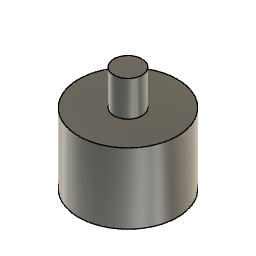
assembly v2 (Autodesk Fusion 360 archive; units mm, degrees)
design "motor1"
Autodesk Fusion 360 part; units mm, degrees
sketch "Sketch1" plane through (0, 0, 0) normal (0, 0, 1) x (1, 0, 0)
  circle A0 centre (0, 0) radius 35
  dimension "d1" = 70
  constraint coincident A0.centre origin
  measures "d1" diameter of A0
extrude "Extrude1" add sketch "Sketch1" along normal blind 50
sketch "Sketch2" plane through (0, 0, 50) normal (0, 0, 1) x (-1, 0, 0)
  circle A0 centre (0, 0) radius 35
  circle A1 centre (0, 0) radius 10
  dimension "d4" = 20
  constraint coincident A0.centre A1.centre
  measures "d4" diameter of A1
extrude "Extrude2" add sketch "Sketch2" along normal blind 25 contours A1

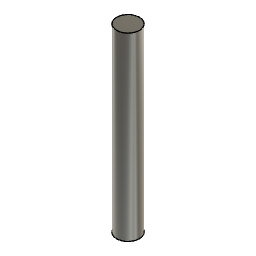
design "crod1"
Autodesk Fusion 360 part; units mm, degrees
sketch "Sketch1" plane through (0, 0, 0) normal (0, 0, 1) x (1, 0, 0)
  circle A0 centre (-0.4902, 0) radius 3
  dimension "d1" = 6
  measures "d1" diameter of A0
extrude "Extrude1" add sketch "Sketch1" along normal blind 47.5

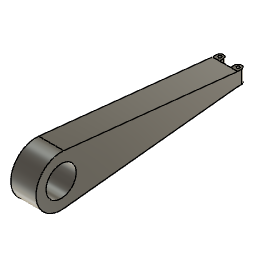
design "arm2"
Autodesk Fusion 360 part; units mm, degrees
sketch "Sketch1" plane through (0, 0, 0) normal (1, 0, 0) x (0, 1, 0)
  circle A0 centre (0, 0) radius 30
  line L0 (5.2264, 49.7261) -> (351.0282, 13.3809)
  line L1 (5.2991, -49.7184) -> (351.0282, -12.87)
  line L2 (351.0282, 13.3809) -> (351.0282, -12.87)
  arc A1 (5.2264, 49.7261) -> (5.2991, -49.7184) centre (0, 0) ccw
  dimension "d1" = 100
  dimension "d2" = 60
  constraint coincident A0.centre A1.centre
  constraint tangent L0 A1
  constraint vertical L2
  measures "d1" diameter of A1
  measures "d2" diameter of A0
extrude "Extrude1" add sketch "Sketch1" along normal blind 50
sketch "Sketch2" plane through (0, 0, 0) normal (0, 0, 1) x (1, 0, 0)
  line L0 (50, 351) -> (36, 351)
  line L1 (36, 351) -> (36, 359)
  line L2 (50, 359) -> (50, 351)
  circle A0 centre (43, 359) radius 3
  line L3 (0, 351) -> (14, 351)
  line L4 (14, 351) -> (14, 359)
  line L5 (0, 359) -> (0, 351)
  circle A1 centre (7, 359) radius 3
  arc A2 (50, 359) -> (36, 359) centre (43, 359) ccw
  arc A3 (14, 359) -> (0, 359) centre (7, 359) ccw
  dimension "d9" = 6
  dimension "d12" = 6
  constraint horizontal L0
  constraint vertical L1
  constraint vertical L2
  constraint concentric A0 A2
  constraint horizontal L3
  constraint vertical L4
  constraint vertical L5
  constraint concentric A1 A3
  measures "d9" diameter of A0
  measures "d12" diameter of A1
extrude "Extrude2" add sketch "Sketch2" along normal blind 13.355 and the other way blind 13.1255
equation "d13 = ( 26.71 / 2 ) * 1 mm"
equation "d15 = ( 26.251 / 2 ) * 1 mm"

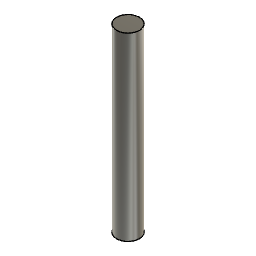
design "crod2"
Autodesk Fusion 360 part; units mm, degrees
sketch "Sketch1" plane through (0, 0, 0) normal (0, 0, 1) x (1, 0, 0)
  circle A0 centre (0, 0) radius 3
  dimension "d1" = 6
  constraint coincident A0.centre origin
  measures "d1" diameter of A0
extrude "Extrude1" add sketch "Sketch1" along normal blind 47.5

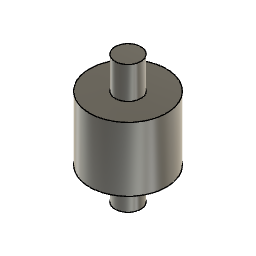
design "motor3"
Autodesk Fusion 360 part; units mm, degrees
sketch "Sketch1" plane through (0, 0, 0) normal (0, 0, 1) x (1, 0, 0)
  circle A0 centre (0, 0) radius 30
  dimension "d1" = 60
  constraint coincident A0.centre origin
  measures "d1" diameter of A0
extrude "Extrude1" add sketch "Sketch1" along normal blind 25
sketch "Sketch2" plane through (0, 0, 25) normal (0, 0, 1) x (-1, 0, 0)
  circle A0 centre (0, 0) radius 30
  circle A1 centre (0, 0) radius 10
  dimension "d4" = 20
  constraint coincident A0.centre A1.centre
  measures "d4" diameter of A1
extrude "Extrude2" add sketch "Sketch2" along normal blind 25 contours A1
mirror "Mirror1" about plane through (0, 0, 0) normal (0, 0, 1) of bodies 1 merged

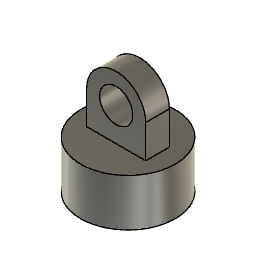
design "base2"
Autodesk Fusion 360 part; units mm, degrees
sketch "Sketch1" plane through (0, 0, 0) normal (0, 0, 1) x (1, 0, 0)
  circle A0 centre (0, 0) radius 100
  dimension "d1" = 200
  constraint coincident A0.centre origin
  measures "d1" diameter of A0
extrude "Extrude1" add sketch "Sketch1" along normal blind 100
sketch "Sketch2" plane through (0, 0, 0) normal (0, 0, -1) x (1, 0, 0)
  circle A0 centre (0, 0) radius 100
  circle A1 centre (0, 0) radius 10
  dimension "d4" = 20
  constraint coincident A0.centre A1.centre
  measures "d4" diameter of A1
extrude "Extrude2" cut sketch "Sketch2" against normal blind 25 contours A1
sketch "Sketch3" plane through (0, 0, 0) normal (0, 1, 0) x (1, 0, 0)
  circle A0 centre (0, -170) radius 35
  line L0 (-62.5, -170) -> (-62.5, -100)
  line L1 (-62.5, -100) -> (62.5, -100)
  line L2 (62.5, -170) -> (62.5, -100)
  arc A1 (-62.5, -170) -> (62.5, -170) centre (0, -170) ccw
  dimension "d7" = 70
  dimension "d8" = 125
  dimension "d9" = 125
  constraint concentric A0 A1
  constraint tangent L0 A1
  constraint vertical L0
  constraint perpendicular L0 L1
  constraint tangent L2 A1
  measures "d7" diameter of A0
  measures "d8" diameter of A1
  measures "d9" distance of L0.end L1.end
extrude "Extrude3" add sketch "Sketch3" along normal mid plane 50

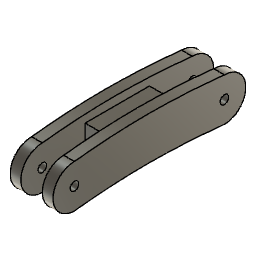
design "arm1"
Autodesk Fusion 360 part; units mm, degrees
sketch "Sketch1" plane through (0, 0, 0) normal (1, 0, 0) x (0, 1, 0)
  spline S0 degree 5 poles (0, 50) (6.8077, 50.7622) (20.44, 52.2195) (40.9391, 54.2045) (68.3744, 56.4426) (102.852, 58.5132) (137.5289, 59.7935) (172.421, 60.2212) (207.5356, 59.7669) (242.8628, 58.4704) (278.3858, 56.3974) (306.9479, 54.1699) (328.445, 52.1996) (342.8095, 50.755) (350, 50) knots 0 0 0 0 0 0 0.1 0.2 0.3 0.4 0.5 0.6 0.7 0.8 0.9 1 1 1 1 1 1
  spline S1 degree 5 poles (0, -50) (6.8077, -49.2378) (20.44, -47.7805) (40.9391, -45.7955) (68.3744, -43.5574) (102.852, -41.4868) (137.5289, -40.2065) (172.421, -39.7788) (207.5356, -40.2331) (242.8628, -41.5296) (278.3858, -43.6026) (306.9479, -45.8301) (328.445, -47.8004) (342.8095, -49.245) (350, -50) knots 0 0 0 0 0 0 0.1 0.2 0.3 0.4 0.5 0.6 0.7 0.8 0.9 1 1 1 1 1 1
  arc A0 (0, 50) -> (10.7493, -48.8308) centre (0, 0) ccw
  circle A1 centre (0, 0) radius 10
  circle A2 centre (350, 0) radius 10
  arc A3 (339.8569, -48.9604) -> (350, 50) centre (350, 0) ccw
  point P0 (170, 60)
  point P1 (170, -40)
  dimension "d1" = 100
  dimension "d2" = 350
  dimension "d3" = 100
  dimension "d4" = 20
  dimension "d5" = 20
  constraint coincident A0.centre A1.centre
  constraint coincident S1.end A3
  constraint coincident S1 A0.end
  constraint concentric A0 A1
  constraint concentric A2 A3
  constraint coincident S1 A3.start
  measures "d1" diameter of A0
  measures "d2" distance of S0.start S0.end
  measures "d3" distance of S0.start S1.start
  measures "d4" diameter of A1
  measures "d5" diameter of A2
extrude "Extrude1" add sketch "Sketch1" along normal blind 25 contours S0 S1 A0 A3
sketch "Sketch2" plane through (25, 0, 0) normal (1, 0, 0) x (0, 1, 0)
  circle A0 centre (350, 0) radius 10
  circle A1 centre (0, 0) radius 10
  arc A2 (0, 50) -> (0, -50) centre (0, 0) ccw
  spline S0 degree 5 poles (0, -50) (2.1482, -49.7595) (4.2972, -49.5223) (6.4471, -49.2885) (8.5978, -49.058) (10.7493, -48.8308) knots 0 0 0 0 0 0 0.031555 0.031555 0.031555 0.031555 0.031555 0.031555
  spline S1 degree 5 poles (10.7493, -48.8308) (15.4162, -48.3381) (26.9111, -47.1643) (45.2687, -45.446) (70.5503, -43.4268) (102.852, -41.4868) (137.5289, -40.2065) (172.421, -39.7788) (207.5356, -40.2331) (242.8628, -41.5296) (276.3801, -43.4855) (302.9169, -45.5185) (322.3782, -47.2522) (334.703, -48.445) (339.8569, -48.9604) knots 0.031555 0.031555 0.031555 0.031555 0.031555 0.031555 0.1 0.2 0.3 0.4 0.5 0.6 0.7 0.8 0.9 0.971769 0.971769 0.971769 0.971769 0.971769 0.971769
  spline S2 degree 5 poles (339.8569, -48.9604) (341.8842, -49.1631) (343.9121, -49.3684) (345.9408, -49.5763) (347.9701, -49.7868) (350, -50) knots 0.971769 0.971769 0.971769 0.971769 0.971769 0.971769 1 1 1 1 1 1
  arc A3 (350, -50) -> (350, 50) centre (350, 0) ccw
  spline S3 degree 5 poles (350, 50) (342.8095, 50.755) (328.445, 52.1996) (306.9479, 54.1699) (278.3858, 56.3974) (242.8628, 58.4704) (207.5356, 59.7669) (172.421, 60.2212) (137.5289, 59.7935) (102.852, 58.5132) (68.3744, 56.4426) (40.9391, 54.2045) (20.44, 52.2195) (6.8077, 50.7622) (0, 50) knots -1 -1 -1 -1 -1 -1 -0.9 -0.8 -0.7 -0.6 -0.5 -0.4 -0.3 -0.2 -0.1 0 0 0 0 0 0
  line L0 (100, 40) -> (250, 40)
  line L1 (250, 40) -> (250, -20)
  line L2 (250, -20) -> (100, -20)
  line L3 (100, -20) -> (100, 40)
  constraint horizontal L0
  constraint vertical L1
  constraint horizontal L2
  constraint vertical L3
extrude "Extrude2" add sketch "Sketch2" along normal blind 25 contours L0 L1 L2 L3
move_body "Move1" bodies 1 to x (1, 0, 0) y (0, 1, 0) z (0, 0, 1) at (-50, 0, 0)
mirror "Mirror1" about plane through (0, 0, 0) normal (1, 0, 0) of bodies 1 merged

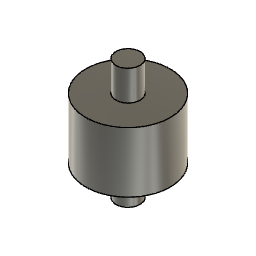
design "motor2"
Autodesk Fusion 360 part; units mm, degrees
sketch "Sketch1" plane through (0, 0, 0) normal (0, 0, 1) x (1, 0, 0)
  circle A0 centre (0, 0) radius 35
  dimension "d1" = 70
  constraint coincident A0.centre origin
  measures "d1" diameter of A0
extrude "Extrude1" add sketch "Sketch1" along normal blind 25
sketch "Sketch2" plane through (0, 0, 25) normal (0, 0, 1) x (-1, 0, 0)
  circle A0 centre (0, 0) radius 35
  circle A1 centre (0, 0) radius 10
  dimension "d4" = 20
  constraint concentric A0 A1
  measures "d4" diameter of A1
extrude "Extrude2" add sketch "Sketch2" along normal blind 25 contours A1
mirror "Mirror1" about plane through (0, 0, 0) normal (0, 0, 1) of bodies 1 merged

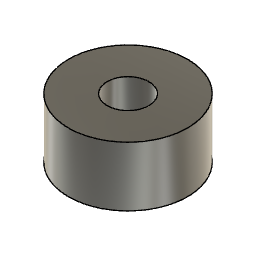
design "base1"
Autodesk Fusion 360 part; units mm, degrees
sketch "Sketch1" plane through (0, 0, 0) normal (0, 0, 1) x (1, 0, 0)
  circle A0 centre (0, 0) radius 100
  dimension "d1" = 200
  constraint coincident A0.centre origin
  measures "d1" diameter of A0
extrude "Extrude1" add sketch "Sketch1" along normal blind 100
sketch "Sketch2" plane through (0, 0, 100) normal (0, 0, 1) x (-1, 0, 0)
  circle A0 centre (0, 0) radius 100
  circle A1 centre (0, 0) radius 35
  dimension "d4" = 70
  constraint coincident A0.centre A1.centre
  measures "d4" diameter of A1
extrude "Extrude2" cut sketch "Sketch2" against normal blind 50 contours A1
